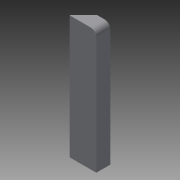
# Autodesk Inventor part: komatex_senzor
Saved by Autodesk Inventor 2015 (Build 190159000, 159)
## iProperties
Created: 2015-01-04
Part Number: komatex_senzor
Material: Generic
Document SubType Name: Modeling
Designer: Turboslimak
Density: 1 g/cm^3
Appearance: Default
Author: Turboslimak
Autodesk Inventor part; units mm, degrees
ref_plane "YZ Plane" through (0, 0, 0) normal (1, 0, 0) x (0, 1, 0)
ref_plane "XZ Plane" through (0, 0, 0) normal (0, 1, 0) x (-1, 0, 0)
ref_plane "XY Plane" through (0, 0, 0) normal (0, 0, 1) x (1, 0, 0)
sketch "Sketch1" plane through (0, 0, 0) normal (0, 1, 0) x (-1, 0, 0)
  line L0 (9.5, -44) -> (-9.5, -44)
  line L1 (-9.5, -44) -> (-9.5, 44)
  line L2 (-9.5, 44) -> (9.5, 44)
  line L3 (9.5, 44) -> (9.5, -44)
  line L4 (9.5, -44) -> (-9.5, 44) construction
  line L5 (-9.5, -44) -> (9.5, 44) construction
  point P0 (0, 0)
  dimension "d0" = 19
  dimension "d1" = 88
  constraints: 12 end point, 2 midpoint, 2 parallel, 1 horizontal, 1 perpendicular
  measures "d0" distance of L1.end L2.end
  measures "d1" distance of L0.end L1.end
extrude "Extrusion1" add sketch "Sketch1" along normal blind 10
fillet "Fillet1" radius 4 1 edges at (9.5, 5, 44)
chamfer "Chamfer1" distance 9.5 angle 45 1 edges at (-9.5, 10, 0)
body "Solid1"
